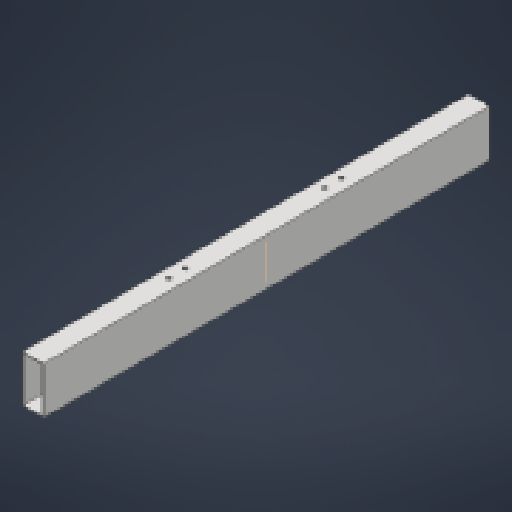
# Autodesk Inventor part: 321x30
Saved by Autodesk Inventor 2025 (Build 290162000, 162)
## iProperties
Created: 2025-11-08
Part Number: 321x30
Material: 常规
Document SubType Name: Modeling
Designer: XH
Density: 1 g/cm^3
Appearance: 默认
Author: XH
Autodesk Inventor part; units mm, degrees
ref_plane "YZ Plane" through (0, 0, 0) normal (1, 0, 0) x (0, 1, 0)
ref_plane "XZ Plane" through (0, 0, 0) normal (0, 1, 0) x (-1, 0, 0)
ref_plane "XY Plane" through (0, 0, 0) normal (0, 0, 1) x (1, 0, 0)
sketch "草图1" plane through (0, 0, 0) normal (0, 0, 1) x (1, 0, 0)
  line L0 (10, -22.5) -> (-10, -22.5)
  line L1 (-10, -22.5) -> (-10, 22.5)
  line L2 (-10, 22.5) -> (10, 22.5)
  line L3 (10, 22.5) -> (10, -22.5)
  line L4 (10, -22.5) -> (-10, 22.5) construction
  line L5 (-10, -22.5) -> (10, 22.5) construction
  line L6 (9, 21.5) -> (-9, 21.5)
  line L7 (-9, 21.5) -> (-9, -21.5)
  line L8 (-9, -21.5) -> (9, -21.5)
  line L9 (9, -21.5) -> (9, 21.5)
  point P0 (0, 0)
  dimension "d0" = 45
  dimension "d1" = 20
  dimension "d4" = 1
  constraints: 20 end point, 4 parallel, 2 midpoint, 2 perpendicular, 1 horizontal, 3 other
  measures "d0" distance of L0.end L1.end
  measures "d1" distance of L0.start L0.end
  measures "d4" distance between parallel lines of L2 L6
extrude "拉伸1" add sketch "草图1" along normal blind 328
sketch "草图4" plane through (-10, 22.5, 0) normal (0, 1, 0) x (1, 0, 0)
  circle A0 centre (9, -81) radius 2
  circle A1 centre (9, -97) radius 2
  line L0 (0, 0) -> (0, -328) projected
  line L1 (20, 0) -> (0, 0) projected
  line L2 (0, -164) -> (-22.908, -164)
  circle A2 centre (9, -247) radius 2
  circle A3 centre (9, -231) radius 2
  point P0 (10, 0)
  dimension "d5" = 9
  dimension "d6" = 16
  dimension "d7" = 81
  constraints: 4 centre point, 2 end point, 2 symmetric about line, 1 horizontal, 1 midpoint, 1 vertical alignment, 2 other
  measures "d5" distance from line of L0 A1.centre
  measures "d6" distance of A1.centre A0.centre
  measures "d7" distance from line of A0.centre L1
extrude "拉伸2" cut sketch "草图4" against normal blind 58.75
sketch "草图5" plane through (0, 0, 328) normal (0, 0, 1) x (1, 0, 0)
  line L0 (10, 22.5) -> (-10, 22.5) projected
  line L1 (-10, 22.5) -> (-10, -22.5) projected
  line L2 (-10, -22.5) -> (10, -22.5) projected
  line L3 (10, -22.5) -> (10, 22.5) projected
  line L4 (9, 21.5) -> (9, -21.5) projected
  line L5 (9, -21.5) -> (-9, -21.5) projected
  line L6 (-9, -21.5) -> (-9, 21.5) projected
  line L7 (-9, 21.5) -> (9, 21.5) projected
  point P0 (0, 0)
ref_plane "工作平面1" through (0, 0, 164) normal (0, 0, 1) x (1, 0, 0)
extrude "拉伸3" add sketch "草图5" along normal blind 50
mirror "镜像1" about plane through (0, 0, 164) normal (0, 0, 1) of "拉伸3"
